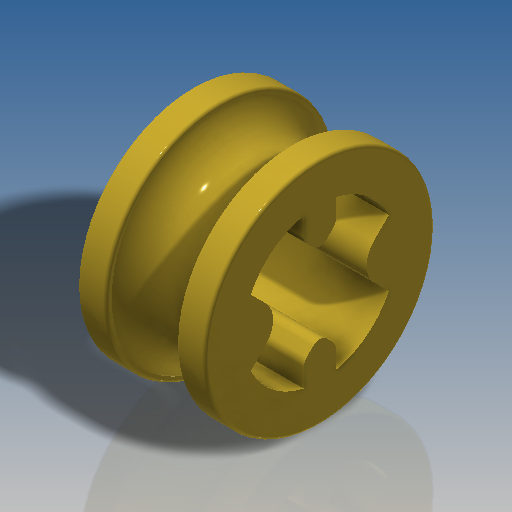
# Autodesk Inventor part: 4265c-Yellow
Saved by Autodesk Inventor 2019.4 (Build 234330000, 330)
## iProperties
Company: Allseas Engineering BV
Created: 2011-12-01
Part Number: 4265c-Yellow
Cost Center: 0 kg
Material: ABS Plastic
Document SubType Name: Modeling
Designer: D. Kohfeld
Authority: 0 mm^3
Mass: 0.0816713 g
Surface Area: 2.27874 cm^2
Volume: 0.0770484 cm^3
Density: 1.06 g/cm^3
Appearance: Yellow
Act. Code: DW000
SaveDate: 2011-07-28
SaveTime: 18:32
FileName: Standard
TotalMass: 0 kg
TotalVolume: 0 mm^3
Subject: =<Title><TITLE 1_2> <TITLE 2_2>
Author: D. Kohfeld
Autodesk Inventor part; units mm, degrees
ref_plane "YZ Plane" through (0, 0, 0) normal (1, 0, 0) x (0, 1, 0)
ref_plane "XZ Plane" through (0, 0, 0) normal (0, 1, 0) x (-1, 0, 0)
ref_plane "XY Plane" through (0, 0, 0) normal (0, 0, 1) x (1, 0, 0)
sketch "Sketch1" plane through (0, 0, 0) normal (0, 0, 1) x (1, 0, 0)
  line L0 (-2, 0) -> (2, 0)
  line L1 (-2, 0) -> (-2, 2.7)
  line L2 (-2, 2.7) -> (-2, 2.7)
  line L3 (0, 0) -> (0, 2.7) construction
  line L4 (-2, 2.7) -> (-2, 3.5)
  line L5 (-1.9, 3.6) -> (-1.2, 3.6)
  line L6 (-2, 2.7) -> (0, 2.7) construction
  arc A0 (-1.1, 3.5) -> (-1.2, 3.6) centre (-1.2, 3.5) ccw
  arc A1 (-1.9, 3.6) -> (-2, 3.5) centre (-1.9, 3.5) ccw
  line L7 (2, 0) -> (2, 2.7)
  line L8 (2, 2.7) -> (2, 2.7)
  line L9 (2, 2.7) -> (2, 3.5)
  line L10 (1.9, 3.6) -> (1.2, 3.6)
  arc A2 (1.2, 3.6) -> (1.1, 3.5) centre (1.2, 3.5) ccw
  arc A3 (2, 3.5) -> (1.9, 3.6) centre (1.9, 3.5) ccw
  line L11 (1.1, 3.5) -> (1.1, 3.4204)
  line L12 (-1.1, 3.5) -> (-1.1, 3.4204)
  arc A4 (-1.1, 3.4204) -> (1.1, 3.4204) centre (0, 3.9) ccw
  dimension "d0" = 0.1
  dimension "d1" = 7.2
  dimension "d2" = 5.4
  dimension "d3" = 5.4
  dimension "d4" = 4
  dimension "d5" = 4
  dimension "d26" = 2.2
  dimension "d27" = 1.2
  constraints: 26 end point, 10 point on circle, 8 symmetric about line, 5 centre point, 5 tangent, 4 perpendicular, 3 parallel, 2 horizontal, 1 coincident, 1 equal radius, 1 midpoint, 1 point on line, 1 vertical, 2 other
  measures "d0" radius of A0
  measures "d1" diameter of L5 L0
  measures "d2" diameter of L6 L0
  measures "d3" diameter of L2 L0
  measures "d4" distance of L0.start L0.end
  measures "d5" distance between parallel lines of L9 L4
  measures "d26" distance between parallel lines of L12 L11
  measures "d27" radius of A4
revolve "Revolution1" add sketch "Sketch1" angle 360 about axis through (-2, 0, 0) along (1, 0, 0)
sketch "Sketch2" plane through (2, 0, 0) normal (1, 0, 0) x (0, 0, -1)
  circle A0 centre (0, 0) radius 2.4
  line L0 (2.1657, -1.0343) -> (1.6314, -0.5) construction
  line L1 (1.1314, 0) -> (1.6314, 0.5)
  line L2 (-2.1657, 1.0343) -> (-1.6314, 0.5) construction
  line L3 (-1.1314, 0) -> (-1.6314, -0.5)
  line L4 (-1.0343, -2.1657) -> (0, -1.1314)
  line L5 (0, -1.1314) -> (1.0343, -2.1657)
  line L6 (1.0343, 2.1657) -> (0, 1.1314)
  line L7 (0, 1.1314) -> (-1.0343, 2.1657)
  line L8 (-1.6314, -0.5) -> (-2.3473, -0.5)
  line L9 (-1.6314, 0.5) -> (-2.3473, 0.5)
  line L10 (1.6314, -0.5) -> (2.3473, -0.5)
  line L11 (1.6314, 0.5) -> (2.3473, 0.5)
  line L12 (-1.6314, -0.5) -> (-2.1657, -1.0343) construction
  line L13 (1.6314, -0.5) -> (1.1314, 0)
  line L14 (1.6314, 0.5) -> (2.1657, 1.0343) construction
  line L15 (-1.6314, 0.5) -> (-1.1314, 0)
  circle A1 centre (0, 0) radius 3.5 projected
  dimension "d11" = 4.8
  dimension "d12" = 1.6
  dimension "d13" = 1
  dimension "d14" = 1
  dimension "d15" = 1.4627
  dimension "d16" = 1.4627
  dimension "d17" = 1.6
  dimension "d18" = 1.6
  dimension "d19" = 1.6
  constraints: 32 end point, 11 perpendicular, 5 equal length, 5 parallel, 2 coincident, 2 collinear, 1 horizontal, 1 vertical alignment, 14 other
  measures "d12" distance between parallel lines of L2 L7
  measures "d13" distance between parallel lines of L9 L8
  measures "d14" distance between parallel lines of L11 L10
  measures "d15" distance of L4.start L4.end
  measures "d16" distance of L12.end L3.start
  measures "d17" distance between parallel lines of L6 L14
  measures "d18" distance between parallel lines of L5 L0
  measures "d19" distance between parallel lines of L12 L4
extrude "Extrusion1" cut sketch "Sketch2" against normal through all contours L11 L1 L13 L10 A0 L5 L4 L8 L3 L15 L9 L7 L6
fillet "Fillet1" radius 0.3 6 edges at (0, 0, 1.1314) (0, 0.5, 1.6314) (0, -0.5, 1.6314) (0, 0.5, -1.6314) (0, 0, -1.1314) (0, -0.5, -1.6314)
fillet "Fillet2" radius 0.8 2 edges at (0, -1.1314, 0) (0, 1.1314, 0)
equation "\"d0\" = lf"
equation "\"d1\" = tlad"
equation "\"d3\" = d2"
equation "\"d4\" = d5"
equation "\"d5\" = 0.5 * lu"
equation "\"d11\" = kd"
equation "\"d12\" = d19"
equation "\"d14\" = d13"
equation "\"d16\" = d15"
equation "\"d17\" = d19"
equation "\"d18\" = d19"
equation "\"d19\" = axlet"
equation "\"lf\" = 0.1"
equation "\"tlad\" = 7.2"
equation "\"lu\" = 8"
equation "\"kd\" = 4.8"
equation "\"axlet\" = 1.6"
body "Solid1"
